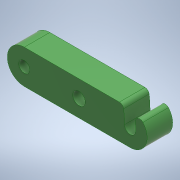
# Autodesk Inventor part: 071_0100_Base
Saved by Autodesk Inventor 2020 (Build 240168000, 168)
## iProperties
Created: 2018-07-06
Part Number: 071_0100_Base
Material: Generic
Document SubType Name: Modeling
Designer: deniz
Density: 1 g/cm^3
Appearance: Default
Author: deniz
Autodesk Inventor part; units mm, degrees
ref_plane "YZ Plane" through (0, 0, 0) normal (1, 0, 0) x (0, 1, 0)
ref_plane "XZ Plane" through (0, 0, 0) normal (0, 1, 0) x (-1, 0, 0)
ref_plane "XY Plane" through (0, 0, 0) normal (0, 0, 1) x (1, 0, 0)
sketch "Sketch1" plane through (0, 0, 0) normal (0, 1, 0) x (-1, 0, 0)
  line L0 (0, 0) -> (-49.7803, 0) construction
  line L1 (0, -8) -> (-49.7803, -8)
  line L2 (-49.7803, 8) -> (0, 8)
  arc A0 (0, -8) -> (0, 8) centre (0, 0) ccw
  arc A1 (-49.7803, 8) -> (-49.7803, -8) centre (-49.7803, 0) ccw
  circle A2 centre (0, 0) radius 2.6
  arc A3 (-49.1333, 8) -> (-49.7803, 0) centre (0, 0) ccw construction
  arc A4 (-51.7488, 8.4259) -> (-52.4303, 0) centre (0, 0) ccw
  arc A5 (-46.5177, 7.5741) -> (-47.1303, 0) centre (0, 0) ccw
  arc A6 (-46.5177, 7.5741) -> (-51.7488, 8.4259) centre (-49.1333, 8) ccw
  arc A7 (-52.4303, 0) -> (-47.1303, 0) centre (-49.7803, 0) ccw
  circle A8 centre (-25.7387, 0) radius 2.95
  circle A9 centre (-25.7387, 0) radius 6
  point P0 (-24.8902, 0)
  dimension "d8" = 49.7803
  dimension "d9" = 5.2
  dimension "d10" = 16
  dimension "d11" = 5.3
  dimension "d12" = 5.9
  dimension "d13" = 25.7387
  dimension "d18" = 12
  constraints: 14 point on circle, 10 centre point, 8 end point, 8 tangent, 3 coincident, 2 point on line, 1 horizontal, 1 midpoint, 1 parallel
  measures "d8" distance of L0.start L0.end
  measures "d9" diameter of A2
  measures "d10" distance between parallel lines of L1 L2
  measures "d11" diameter of A6
  measures "d12" diameter of A8
  measures "d13" distance of L0.start A8.centre
  measures "d18" diameter of A9
extrude "Extrusion3" add sketch "Sketch1" along normal blind 4 contours L1 A1 A4 A7 A5 A6 L2 A0 | A1 L2 A6 A5 A7 A4 | A9
extrude "Extrusion4" cut sketch "Sketch1" along normal blind 10 contours A4 A6 L2 A1 | A1 L2 A6 A5 A7 A4
extrude "Extrusion5" [suppressed]
move faces "Move1" translate (0, -8, 0) faces at (25.0545, 0, -6.3095)
fillet "Fillet2" radius 2 2 edges at (46.4833, -2, 8) (51.858, -2, 7.7255)
equation "\"d8\" = d_clamp_total"
equation "\"d13\" = d_clamp_center"
equation "\"d_clamp_total\" = 49.780317"
equation "\"d_clamp_center\" = 25.738687"
body "Solid2"
